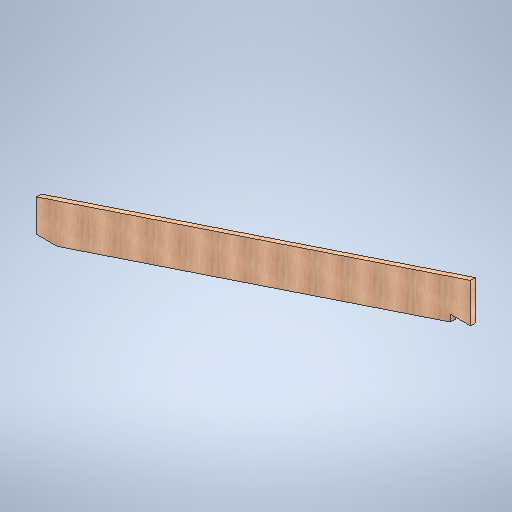
# Autodesk Inventor part: Rafter
Saved by Autodesk Inventor 2025 (Build 290162010, 162A)
## iProperties
Created: 2024-09-15
Part Number: Rafter
Material: Wood (Birch)
Document SubType Name: Modeling
Designer: Tom
Density: 0.55 g/cm^3
Appearance: Birch - Natural Polished
Author: Tom
Autodesk Inventor part; units mm, degrees
ref_plane "YZ Plane" through (0, 0, 0) normal (1, 0, 0) x (0, 1, 0)
ref_plane "XZ Plane" through (0, 0, 0) normal (0, 1, 0) x (-1, 0, 0)
ref_plane "XY Plane" through (0, 0, 0) normal (0, 0, 1) x (1, 0, 0)
sketch "Sketch1" plane through (0, 0, 0) normal (0, 0, 1) x (1, 0, 0)
  line L0 (0, 0) -> (3230.5625, 1076.8542)
  line L1 (3230.5625, 1384.7546) -> (-161.925, 253.9254)
  line L2 (0, 0) -> (-161.925, 0)
  line L3 (-161.925, 0) -> (-161.925, 253.9254)
  line L4 (1454.7512, 484.9171) -> (1454.7512, 586.5171)
  line L5 (1454.7512, 586.5171) -> (1759.5512, 586.5171)
  line L6 (-161.925, 253.9254) -> (1499.1178, 807.6064)
  line L7 (3230.5625, 1076.8542) -> (3073.4, 1076.8542)
  line L8 (3073.4, 1076.8542) -> (3073.4, 1024.4667)
  line L9 (3230.5625, 1076.8542) -> (3230.5625, 1384.7546)
  line L10 (-139.7, 0) -> (-139.7, 261.3338)
  line L11 (3213.1, 1076.8542) -> (3213.1, 1378.9338)
  dimension "d5" = 292.1
  dimension "d8" = 101.6
  dimension "d9" = 304.8
  dimension "d12" = 161.925
  dimension "d13" = 157.1625
  dimension "d17" = 139.7
  dimension "d18" = 139.7
  dimension "d19" = 3352.8
  constraints: 24 end point, 7 point on line, 5 vertical, 3 horizontal, 2 coincident, 1 collinear, 1 perpendicular
  measures "d5" distance between parallel lines of L1 L0
  measures "d8" distance of L4.start L4.end
  measures "d9" distance of L4.end L5.end
  measures "d12" distance of L0.start L2.end
  measures "d13" distance of L0.end L7.end
  measures "d17" distance from line of L10 point (0, 0)
  measures "d18" distance from line of L11 L7.end
  measures "d19" distance between parallel lines of L10 L11
extrude "Extrusion1" add sketch "Sketch1" along normal blind 38.1 contours L2 L10 L1 L11 L7 L8 L0 L5 L4 | L4 L5 L0 | L2 L3 L1 L10 | L7 L11 L1 L9
body "Solid1"
